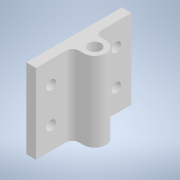
# Autodesk Inventor part: joint_female
Saved by Autodesk Inventor 2020 (Build 240168000, 168)
## iProperties
Created: 2020-05-03
Part Number: joint_female
Material: Generic
Document SubType Name: Modeling
Designer: galaxy
Density: 1 g/cm^3
Appearance: Default
Author: galaxy
Autodesk Inventor part; units mm, degrees
ref_plane "YZ Plane" through (0, 0, 0) normal (1, 0, 0) x (0, 1, 0)
ref_plane "XZ Plane" through (0, 0, 0) normal (0, 1, 0) x (-1, 0, 0)
ref_plane "XY Plane" through (0, 0, 0) normal (0, 0, 1) x (1, 0, 0)
sketch "Sketch1" plane through (0, 0, 0) normal (0, 1, 0) x (-1, 0, 0)
  line L0 (1.5, 15) -> (-1.5, 15)
  line L1 (-1.5, -15) -> (1.5, -15)
  line L2 (1.5, -15) -> (1.5, 15)
  line L3 (1.5, 15) -> (-1.5, -15) construction
  line L4 (-1.5, 15) -> (1.5, -15) construction
  arc A0 (-5, 3.5) -> (-5, -3.5) centre (-5, 0) ccw
  circle A1 centre (-5, 0) radius 2
  line L5 (-5, -3.5) -> (-3.5, -3.5)
  line L6 (-5, 3.5) -> (-3.5, 3.5)
  line L7 (-1.5, 15) -> (-1.5, 5.5)
  line L8 (-1.5, -5.5) -> (-1.5, -15)
  arc A2 (-3.5, 3.5) -> (-1.5, 5.5) centre (-3.5, 5.5) ccw
  arc A3 (-1.5, -5.5) -> (-3.5, -3.5) centre (-3.5, -5.5) ccw
  point P0 (0, 0)
  dimension "d0" = 3
  dimension "d1" = 30
  dimension "d2" = 7
  dimension "d3" = 4
  dimension "d4" = 2
  constraints: 18 end point, 7 tangent, 6 perpendicular, 6 point on circle, 4 centre point, 3 parallel, 2 midpoint, 1 coincident, 1 equal radius, 1 horizontal
  measures "d0" distance of L1.end L1.start
  measures "d1" distance of L1.start L0.end
  measures "d2" diameter of A0
  measures "d3" diameter of A1
  measures "d4" radius of A2
extrude "Extrusion1" add sketch "Sketch1" along normal blind 25
sketch "Sketch2" plane through (1.5, 0, 15) normal (1, 0, 0) x (0, 0, -1)
  circle A0 centre (4.75, 18) radius 1.5
  circle A1 centre (4.75, 7) radius 1.5
  line L0 (0, 0) -> (0, 25) projected
  line L1 (0, 25) -> (9.5, 25) projected
  line L2 (0, 0) -> (9.5, 0) projected
  point P0 (15, 0)
  dimension "d7" = 3
  dimension "d8" = 3
  dimension "d9" = 4.75
  dimension "d10" = 4.75
  dimension "d11" = 7
  dimension "d15" = 7
  constraints: 2 centre point
  measures "d7" diameter of A0
  measures "d8" diameter of A1
  measures "d9" distance from line of L0 A0.centre
  measures "d10" distance from line of L0 A1.centre
  measures "d11" distance from line of L1 A0.centre
  measures "d15" distance from line of L2 A1.centre
extrude "Extrusion2" cut sketch "Sketch2" against normal blind 25
mirror "Mirror1" about plane through (0, 0, 0) normal (0, 0, 1) of "Extrusion2"
body "Solid1"
